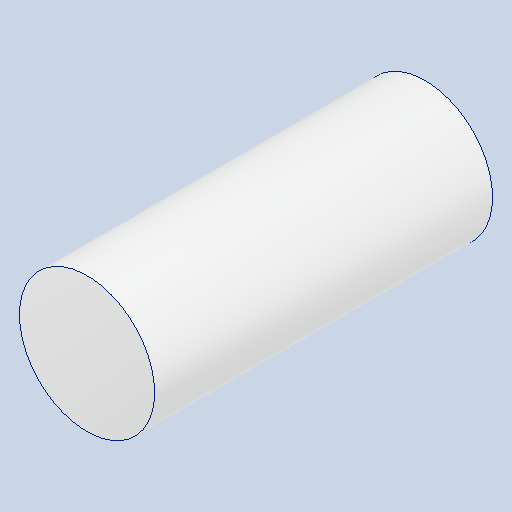
# Autodesk Inventor part: 볼트M4 10mm
Saved by Autodesk Inventor 2024 (Build 280153000, 153)
## iProperties
Created: 2024-04-15
Part Number: 볼트M4 10mm
Material: 알루미늄 6061
Document SubType Name: Modeling
Designer: kkamin5
Density: 2.7 g/cm^3
Appearance: 알루미늄 - 평지
Mass: 0.339292 g
Surface Area: 1.50796 cm^2
Volume: 0.125664 cm^3
Author: kkamin5
Autodesk Inventor part; units mm, degrees
ref_plane "YZ Plane" through (0, 0, 0) normal (1, 0, 0) x (0, 1, 0)
ref_plane "XZ Plane" through (0, 0, 0) normal (0, 1, 0) x (-1, 0, 0)
ref_plane "XY Plane" through (0, 0, 0) normal (0, 0, 1) x (1, 0, 0)
sketch "스케치1" plane through (0, 0, 0) normal (0, 0, 1) x (1, 0, 0)
  circle A0 centre (0, 0) radius 2
  dimension "d0" = 4
  constraints: 1 centre point, 1 coincident
  measures "d0" diameter of A0
extrude "돌출1" add sketch "스케치1" along normal mid plane 10
